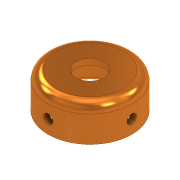
# Autodesk Inventor part: ToolCap
Saved by Autodesk Inventor 2021 (Build 250183000, 183)
## iProperties
Created: 2022-08-25
Part Number: ToolCap
Material: PC/ABS Plastic
Document SubType Name: Modeling
Designer: brian
Density: 0.357273 g/cm^3
Appearance: Metal 1600F Hot
Mass: 0.995214 g
Surface Area: 28.8949 cm^2
Volume: 2.78559 cm^3
Author: brian
## iProperties of the stored document _3DPrint.ipt
Created: 2022-08-26
Part Number: _3DPrint
Material: Generic
Document SubType Name: Modeling
Designer: brian
Density: 1 g/cm^3
Appearance: Default
Author: brian
Autodesk Inventor part; units mm, degrees
ref_plane "YZ Plane" through (0, 0, 0) normal (1, 0, 0) x (0, 1, 0)
ref_plane "XZ Plane" through (0, 0, 0) normal (0, 1, 0) x (-1, 0, 0)
ref_plane "XY Plane" through (0, 0, 0) normal (0, 0, 1) x (1, 0, 0)
sketch "Sketch1" plane through (0, 0, 0) normal (0, 1, 0) x (-1, 0, 0)
  circle A0 centre (0, 0) radius 12.35
  circle A1 centre (0, 0) radius 5
  circle A2 centre (0, 0) radius 14.35
  dimension "d0" = 24.7
  dimension "d1" = 10
  dimension "d2" = 28.7
  constraints: 3 centre point, 3 coincident
  measures "d0" diameter of A0
  measures "d1" diameter of A1
  measures "d2" diameter of A2
extrude "Extrusion1" add sketch "Sketch1" along normal blind 10 contours A2
sketch "Sketch2" plane through (0, 10, 0) normal (0, 1, 0) x (1, 0, 0)
  circle A0 centre (0, 0) radius 14.35 projected
  circle A1 centre (0, 0) radius 4.75
  dimension "d5" = 9.5
  constraints: 1 centre point, 1 coincident
  measures "d5" diameter of A1
extrude "Extrusion2" add sketch "Sketch2" along normal blind 2
fillet "Fillet1" radius 3 2 edges at (12.35, 10, 0) (-14.35, 12, 0)
sketch "Sketch3" plane through (0, 0, 0) normal (0, -1, 0) x (1, 0, 0)
  line L0 (1.5, 12.35) -> (-1.5, 12.35)
  line L1 (-1.5, 12.35) -> (-1.5, 11.35)
  line L2 (-0.5, 10.35) -> (0.5, 10.35)
  line L3 (1.5, 11.35) -> (1.5, 12.35)
  circle A0 centre (0, 0) radius 14.35 projected
  circle A1 centre (0, 0) radius 12.35 projected
  arc A2 (0.5, 10.35) -> (1.5, 11.35) centre (0.5, 11.35) ccw
  arc A3 (-1.5, 11.35) -> (-0.5, 10.35) centre (-0.5, 11.35) ccw
  line L4 (-12.35, 1.5) -> (-12.35, -1.5)
  line L5 (-12.35, -1.5) -> (-11.35, -1.5)
  line L6 (-10.35, -0.5) -> (-10.35, 0.5)
  line L7 (-11.35, 1.5) -> (-12.35, 1.5)
  arc A4 (-10.35, 0.5) -> (-11.35, 1.5) centre (-11.35, 0.5) ccw
  arc A5 (-11.35, -1.5) -> (-10.35, -0.5) centre (-11.35, -0.5) ccw
  line L8 (-1.5, -12.35) -> (1.5, -12.35)
  line L9 (1.5, -12.35) -> (1.5, -11.35)
  line L10 (0.5, -10.35) -> (-0.5, -10.35)
  line L11 (-1.5, -11.35) -> (-1.5, -12.35)
  arc A6 (-0.5, -10.35) -> (-1.5, -11.35) centre (-0.5, -11.35) ccw
  arc A7 (1.5, -11.35) -> (0.5, -10.35) centre (0.5, -11.35) ccw
  line L12 (12.35, -1.5) -> (12.35, 1.5)
  line L13 (12.35, 1.5) -> (11.35, 1.5)
  line L14 (10.35, 0.5) -> (10.35, -0.5)
  line L15 (11.35, -1.5) -> (12.35, -1.5)
  arc A8 (10.35, -0.5) -> (11.35, -1.5) centre (11.35, -0.5) ccw
  arc A9 (11.35, 1.5) -> (10.35, 0.5) centre (11.35, 0.5) ccw
  point P0 (-1.5, 10.35)
  point P1 (1.5, 10.35)
  point P2 (0, 10.35)
  point P3 (-10.35, -1.5)
  point P4 (-10.35, 1.5)
  point P5 (-10.35, 0)
  point P6 (1.5, -10.35)
  point P7 (-1.5, -10.35)
  point P8 (0, -10.35)
  point P9 (10.35, 1.5)
  point P10 (10.35, -1.5)
  point P11 (10.35, 0)
  point P12 (1.5, 12.2586)
  point P13 (-1.5, 12.2586)
  point P14 (-1.5, -12.2586)
  point P15 (1.5, -12.2586)
  point P16 (12.2586, -1.5)
  point P17 (12.2586, 1.5)
  dimension "d9" = 3
  dimension "d10" = 2
  dimension "d11" = 1
  dimension "d14" = 360
  constraints: 32 end point, 16 point on circle, 16 point on line, 8 centre point, 5 tangent, 2 parallel, 1 equal radius, 1 horizontal, 1 midpoint, 1 perpendicular, 1 vertical alignment, 69 other
  measures "d9" distance of point (-1.5, 10.35) point (1.5, 10.35)
  measures "d10" distance of point (1.5, 10.35) L0.start
  measures "d11" radius of A2
extrude "Extrusion3" add sketch "Sketch3" against normal blind 3 contours A1 L3 A2 L2 A3 L1 | A1 L15 A8 L14 A9 L13 | L7 A4 L6 A5 L5 A1 | A1 L4 L7 | A1 L5 L4 | A1 L11 A6 L10 A7 L9
fillet "Fillet2" radius 1 44 edges at (-11.8043, 0, -1.5) (-10.6429, 0, -1.2071) (-10.35, 0, 0) (-10.6429, 0, 1.2071) (-11.8043, 0, 1.5) (-8.7328, 0, 8.7328) (-1.5, 0, 11.8043) (-1.2071, 0, 10.6429) (0, 0, 10.35) (1.2071, 0, 10.6429) (1.5, 0, 11.8043) (8.7328, 0, 8.7328) (11.8043, 0, 1.5) (10.6429, 0, 1.2071) (10.35, 0, 0) (10.6429, 0, -1.2071) (11.8043, 0, -1.5) (8.7328, 0, -8.7328) (1.5, 0, -11.8043) (1.2071, 0, -10.6429) (0, 0, -10.35) (-1.2071, 0, -10.6429) (-1.5, 0, -11.8043) (-8.7328, 0, -8.7328) (-1.2071, 3, 10.6429) (-1.5, 3, 11.8043) (0, 3, 10.35) (1.2071, 3, 10.6429) (1.5, 3, 11.8043) (10.6429, 3, -1.2071) (10.35, 3, 0) (10.6429, 3, 1.2071) (11.8043, 3, 1.5) (11.8043, 3, -1.5) (-1.2071, 3, -10.6429) (0, 3, -10.35) (1.2071, 3, -10.6429) (1.5, 3, -11.8043) (-1.5, 3, -11.8043) (-10.6429, 3, 1.2071) (-10.35, 3, 0) (-10.6429, 3, -1.2071) (-11.8043, 3, -1.5) (-11.8043, 3, 1.5)
fillet "Fillet2" radius 0.5 8 edges at (1.5, 1.5, -12.2586) (-1.5, 1.5, -12.2586) (-12.2586, 1.5, 1.5) (-12.2586, 1.5, -1.5) (-1.5, 1.5, 12.2586) (1.5, 1.5, 12.2586) (12.2586, 1.5, -1.5) (12.2586, 1.5, 1.5)
sketch "Sketch4" plane through (0, 0, 0) normal (0, 0, 1) x (1, 0, 0)
  circle A0 centre (0, 4.6) radius 1.6
  point P0 (0, 0)
  dimension "d20" = 3.2
  dimension "d21" = 4.6
  constraints: 1 centre point, 1 vertical alignment
  measures "d20" diameter of A0
  measures "d21" distance of point (0, 0) A0.centre
extrude "Extrusion4" cut sketch "Sketch4" against normal mid plane 40
sketch "Sketch5" plane through (0, 0, 0) normal (1, 0, 0) x (0, 1, 0)
  circle A0 centre (4.6, 0) radius 1.6
  point P0 (0, 0)
  dimension "d24" = 3.2
  dimension "d25" = 4.6
  constraints: 1 centre point, 1 horizontal alignment
  measures "d24" diameter of A0
  measures "d25" distance of point (0, 0) A0.centre
extrude "Extrusion5" cut sketch "Sketch5" along normal mid plane 40
body "Solid1"
